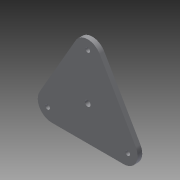
# Autodesk Inventor part: Triangle-5-16-hole
Saved by Autodesk Inventor 2013 (Build 170138000, 138)
## iProperties
Created: 2014-01-31
Part Number: Triangle-5-16-hole
Material: Generic
Document SubType Name: Modeling
Designer: robotics
Density: 1 g/cm^3
Author: robotics
Autodesk Inventor part; units mm, degrees
ref_plane "YZ Plane" through (0, 0, 0) normal (1, 0, 0) x (0, 1, 0)
ref_plane "XZ Plane" through (0, 0, 0) normal (0, 1, 0) x (-1, 0, 0)
ref_plane "XY Plane" through (0, 0, 0) normal (0, 0, 1) x (1, 0, 0)
sketch "Sketch2" plane through (0, 0, 0) normal (0, 0, 1) x (1, 0, 0)
  circle A0 centre (0, 0) radius 3.9688
  circle A1 centre (0, 63.5) radius 3.175
  circle A2 centre (-54.9926, -31.75) radius 3.175
  circle A3 centre (54.9926, -31.75) radius 3.175
  line L0 (0, 69.85) -> (60.4919, -34.925) construction
  line L1 (60.4919, -34.925) -> (-60.4919, -34.925) construction
  line L2 (-60.4919, -34.925) -> (0, 69.85) construction
  line L3 (0, 95.25) -> (82.4889, -47.625)
  line L4 (82.4889, -47.625) -> (-82.4889, -47.625)
  line L5 (-82.4889, -47.625) -> (0, 95.25)
  dimension "d0" = 7.9375
  dimension "d1" = 6.35
  dimension "d2" = 63.5
  dimension "d5" = 360
  dimension "d8" = 12.7
  dimension "d9" = 12.7
  dimension "d10" = 12.7
  constraints: 12 end point, 6 tangent, 4 centre point, 3 parallel, 1 coincident, 1 vertical alignment, 7 other
  measures "d0" diameter of A0
  measures "d1" diameter of A1
  measures "d2" distance of A0.centre A1.centre
  measures "d8" distance between parallel lines of L4 L1
  measures "d9" distance between parallel lines of L5 L2
  measures "d10" distance between parallel lines of L3 L0
extrude "Extrusion1" add sketch "Sketch2" along normal blind 6.35
fillet "Fillet1" radius 19.05 3 edges at (0, 95.25, 3.175) (-82.4889, -47.625, 3.175) (82.4889, -47.625, 3.175)
body "Solid1"
